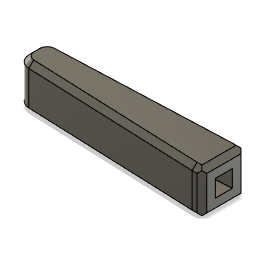
Light Switch Extension Lever v2 (Autodesk Fusion 360 design; units mm, degrees)
Autodesk Fusion 360 part; units mm, degrees
sketch "Sketch1" plane through (0, 0, 0) normal (0, 1, 0) x (1, 0, 0)
  line L0 (0, 0) -> (-78.5, 0)
  line L1 (-78.5, 0) -> (-78.5, 18)
  line L2 (-78.5, 18) -> (0, 18)
  line L3 (0, 18) -> (0, 0)
  line L4 (-4, 18) -> (-78.5, 15)
  line L5 (-4, 0) -> (-78.5, 3)
  dimension "d1" = 78.5
  dimension "d2" = 18
  dimension "d3" = 4
  dimension "d4" = 3
  dimension "d5" = 3
  constraint horizontal L0
  constraint vertical L1
  constraint horizontal L2
  constraint vertical L3
  constraint coincident L0.start L3.end
  constraint coincident L2 L4.start
  constraint coincident L1 L4.end
  constraint coincident L0 L5.start
  constraint coincident L1 L5.end
  constraint vertical L4.start L5.start
  measures "d1" distance of L1.end L2.end
  measures "d2" distance of L0.start L2.end
  measures "d3" distance of L2.end L4.start
  measures "d4" distance of L1.end L4.end
  measures "d5" distance of L0.end L5.end
extrude "Extrude1" add sketch "Sketch1" along normal blind 18 contours L0 L1 L2 L3 L4 L5
sketch "Sketch2" plane through (0, 0, 0) normal (1, 0, 0) x (0, 0, -1)
  line L0 (0, 0) -> (18, 0)
  line L1 (18, 0) -> (18, 18)
  line L2 (18, 18) -> (0, 18)
  line L3 (0, 18) -> (0, 0)
  line L4 (18, 18) -> (0, 0) construction
  line L5 (12.5, 5.5) -> (5.5, 5.5)
  line L6 (5.5, 5.5) -> (5.5, 12.5)
  line L7 (5.5, 12.5) -> (12.5, 12.5)
  line L8 (12.5, 12.5) -> (12.5, 5.5)
  line L9 (12.5, 5.5) -> (5.5, 12.5) construction
  line L10 (5.5, 5.5) -> (12.5, 12.5) construction
  point P0 (9, 9)
  dimension "d8" = 7
  dimension "d9" = 7
  constraint coincident L1.end L2.start
  constraint coincident L0.start L3.end
  constraint horizontal L5
  constraint perpendicular L5 L6
  constraint parallel L5 L7
  constraint parallel L6 L8
  constraint coincident L9 P0
  constraint coincident L10 P0
  constraint midpoint L4 P0
  measures "d8" distance of L6.end L7.end
  measures "d9" distance of L5.start L7.end
extrude "Extrude2" cut sketch "Sketch2" against normal blind 15 contours L5 L6 L7 L8
chamfer "Chamfer1" distance 2 angle 45 4 edges at (0, 18, -9) (0, 9, -18) (0, 9, 0) (0, 0, -9)
fillet "Fillet1" radius 5 2 edges at (-78.5, 9, -3) (-78.5, 9, -15)
chamfer "Chamfer3" distance 2 angle 45 14 edges at (-38.8506, 18, -1.4034) (-38.8506, 18, -16.5966) (-77.106, 18, -13.661) (-78.5, 18, -9) (-77.106, 18, -4.339) (-3, 18, -18) (-3, 18, 0) (-38.8506, 0, -1.4034) (-77.106, 0, -4.339) (-78.5, 0, -9) (-77.106, 0, -13.661) (-38.8506, 0, -16.5966) (-3, 0, -18) (-3, 0, 0)
chamfer "Chamfer4" distance 15 distance2 1 2 edges at (-15, 9, -12.5) (-15, 9, -5.5) measured on face at (-5, 10.1667, -12.5) measured on face at (-5, 7.8333, -5.5)
equation "d8 = Switch_Thickness"
equation "d9 = Switch_Thickness"
equation "Switch_Thickness = 7 mm" comment "Thickness of Light Switch Lever"
